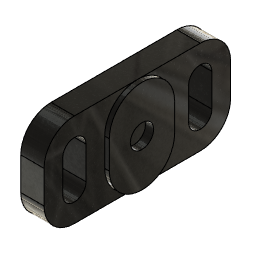
Z Idler Top Front_2x v2 (Autodesk Fusion 360 design; units mm, degrees)
Autodesk Fusion 360 part; units mm, degrees
sketch "Sketch1" plane through (0, 0, 0) normal (1, 0, 0) x (0, 1, 0)
  line L0 (20, -10) -> (-20, -10)
  line L1 (-20, -10) -> (-20, 10)
  line L2 (-20, 10) -> (20, 10)
  line L3 (20, 10) -> (20, -10)
  line L4 (20, -10) -> (-20, 10) construction
  line L5 (-20, -10) -> (20, 10) construction
  line L6 (-13.5, 0) -> (13.5, 0) construction
  line L7 (0, 0) -> (0, 10) construction
  line L8 (7, 10) -> (7, -10)
  line L9 (-7, 10) -> (-7, -10)
  circle A0 centre (0, 0) radius 2.5
  line L10 (11, 3.5) -> (11, -3.5)
  arc A1 (11, -3.5) -> (16, -3.5) centre (13.5, -3.5) ccw
  line L11 (16, -3.5) -> (16, 3.5)
  arc A2 (16, 3.5) -> (11, 3.5) centre (13.5, 3.5) ccw
  line L12 (13.5, 3.5) -> (13.5, -3.5) construction
  line L13 (-11, 3.5) -> (-11, -3.5)
  arc A3 (-16, -3.5) -> (-11, -3.5) centre (-13.5, -3.5) ccw
  line L14 (-16, -3.5) -> (-16, 3.5)
  arc A4 (-11, 3.5) -> (-16, 3.5) centre (-13.5, 3.5) ccw
  point P0 (13.5, 0)
  dimension "d3949" = 40
  dimension "d3950" = 20
  dimension "d3954" = 14
  dimension "d3955" = 5
  dimension "d3956" = 4
  dimension "d3957" = 4
  dimension "d3958" = 5
  constraint horizontal L0
  constraint perpendicular L0 L1
  constraint parallel L0 L2
  constraint parallel L1 L3
  constraint coincident L4 L7.start
  constraint coincident L5 L7.start
  constraint coincident L7.start A0.centre
  constraint horizontal L6
  constraint midpoint L7.start L6
  constraint midpoint L2 L7.end
  constraint coincident L2 L8.start
  constraint coincident L0 L8.end
  constraint perpendicular L0 L8
  constraint symmetric L7 L8.start L9.start
  constraint symmetric L7 L8.end L9.end
  constraint tangent L10 A1
  constraint tangent A1 L11
  constraint parallel L10 L11
  constraint tangent L11 A2
  constraint tangent L10 A2
  constraint perpendicular L6 L12
  constraint coincident P0 L6.end
  constraint midpoint L12 P0
  constraint symmetric L7 L10.start L13.start
  constraint symmetric L7 L10.end L13.end
  constraint symmetric L7 A1.end A3.start
  constraint symmetric L7 L11.end L14.end
  constraint symmetric L7 A1 A3
  constraint symmetric L7 A2 A4
  measures "d3949" distance of L1.end L2.end
  measures "d3950" distance of L0.end L1.end
  measures "d3954" distance of L8 L9
  measures "d3955" diameter of A1
  measures "d3956" distance of L2 A2
  measures "d3957" distance of L3 L11
  measures "d3958" diameter of A0
extrude "Extrude1" add sketch "Sketch1" along normal blind 5 contours L0 L2 L3 L8 | L0 L1 L2 L9 makes body 1 at (0, 18.6667, -1.1667) makes body 2 at (0, -18.6667, -1.1667)
extrude "Extrude2" add sketch "Sketch1" along normal blind 6 contours L0 L2 L8 L9 bodies 1 2
fillet "Fillet1" radius 6.5 4 edges at (2.5, -20, 10) (2.5, 20, 10) (2.5, 20, -10) (2.5, -20, -10) on bodies 1
fillet "Fillet1" radius 7 4 edges at (5.5, -7, 10) (5.5, 7, 10) (5.5, -7, -10) (5.5, 7, -10) on bodies 1
sketch "Sketch2" plane through (0, 0, 0) normal (-1, 0, 0) x (0, -1, 0)
  arc A0 (13.5, -10) -> (20, -3.5) centre (13.5, -3.5) ccw
  line L0 (20, -3.5) -> (20, 3.5)
  arc A1 (20, 3.5) -> (13.5, 10) centre (13.5, 3.5) ccw
  line L1 (13.5, 10) -> (-13.5, 10)
  arc A2 (-13.5, 10) -> (-20, 3.5) centre (-13.5, 3.5) ccw
  line L2 (-20, 3.5) -> (-20, -3.5)
  arc A3 (-20, -3.5) -> (-13.5, -10) centre (-13.5, -3.5) ccw
  line L3 (-13.5, -10) -> (13.5, -10)
  arc A4 (11, -3.5) -> (16, -3.5) centre (13.5, -3.5) ccw
  line L4 (11, -3.5) -> (11, 3.5)
  arc A5 (16, 3.5) -> (11, 3.5) centre (13.5, 3.5) ccw
  line L5 (16, 3.5) -> (16, -3.5)
  circle A6 centre (0, 0) radius 2.5 construction
  arc A7 (-11, 3.5) -> (-16, 3.5) centre (-13.5, 3.5) ccw
  line L6 (-11, 3.5) -> (-11, -3.5)
  arc A8 (-16, -3.5) -> (-11, -3.5) centre (-13.5, -3.5) ccw
  line L7 (-16, -3.5) -> (-16, 3.5)
  circle A9 centre (0, 0) radius 2.5
  line L8 (2.3094, -4) -> (4.6188, 0)
  line L9 (4.6188, 0) -> (2.3094, 4)
  line L10 (2.3094, 4) -> (-2.3094, 4)
  line L11 (-2.3094, 4) -> (-4.6188, 0)
  line L12 (-4.6188, 0) -> (-2.3094, -4)
  line L13 (-2.3094, -4) -> (2.3094, -4)
  dimension "d3969" = 4
  constraint coincident A6.centre A9.centre
  constraint horizontal L13
  measures "d3969" distance of A6.centre L13
extrude "Extrude3" cut sketch "Sketch2" against normal blind 4 contours A9 | L8 L9 L10 L11 L12 L13 bodies 1
sketch "Sketch3" plane through (4, 0, 0) normal (-1, 0, 0) x (0, -1, 0)
  circle A0 centre (0, 0) radius 2.5
  line L0 (-2.3094, -4) -> (2.3094, -4)
  line L1 (2.3094, -4) -> (4.6188, 0)
  line L2 (4.6188, 0) -> (2.3094, 4)
  line L3 (2.3094, 4) -> (-2.3094, 4)
  line L4 (-2.3094, 4) -> (-4.6188, 0)
  line L5 (-4.6188, 0) -> (-2.3094, -4)
  circle A1 centre (0, 0) radius 2.5
extrude "Extrude4" add sketch "Sketch3" against normal blind 0.25 contours A0 A1 bodies 1
named bodies: "Z Idler Top Front Buddy_2x"
